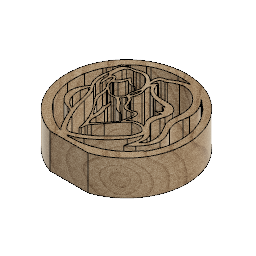
mother's-day-01-v2 (Autodesk Fusion 360 design; units mm, degrees)
Autodesk Fusion 360 part; units mm, degrees
(part 1 of 2)
sketch "Sketch1" plane through (0, 0, 0) normal (0, 0, 1) x (1, 0, 0)
  spline S0 degree 3 poles (69.4054, 110.167) (64.1585, 109.9181) (58.2066, 108.342) (54.0588, 106.0815) knots 0 0 0 0 1 1 1 1
  spline S1 degree 3 poles (54.0588, 106.0815) (53.4367, 105.7289) (52.5034, 105.2312) (51.985, 104.9409) knots 0 0 0 0 1 1 1 1
  spline S2 degree 3 poles (51.985, 104.9409) (49.1438, 103.4062) (45.3279, 100.4198) (45.5145, 99.8599) knots 0 0 0 0 1 1 1 1
  spline S3 degree 3 poles (45.5145, 99.8599) (45.5352, 99.7562) (45.4938, 99.7355) (45.3901, 99.7977) knots 0 0 0 0 1 1 1 1
  spline S4 degree 3 poles (45.3901, 99.7977) (45.2864, 99.8599) (44.9753, 99.6733) (44.7057, 99.3622) knots 0 0 0 0 1 1 1 1
  spline S5 degree 3 poles (44.7057, 99.3622) (44.3117, 98.9267) (44.2909, 98.8437) (44.5813, 98.9474) knots 0 0 0 0 1 1 1 1
  spline S6 degree 3 poles (44.5813, 98.9474) (44.8094, 99.0304) (44.9131, 99.0096) (44.8301, 98.8852) knots 0 0 0 0 1 1 1 1
  spline S7 degree 3 poles (44.8301, 98.8852) (44.7679, 98.7608) (44.5191, 98.6778) (44.2909, 98.6778) knots 0 0 0 0 1 1 1 1
  spline S8 degree 3 poles (44.2909, 98.6778) (43.8554, 98.6778) (43.7517, 98.3667) (44.1665, 98.1801) knots 0 0 0 0 1 1 1 1
  spline S9 degree 3 poles (44.1665, 98.1801) (44.2909, 98.1179) (44.1872, 98.1179) (43.8969, 98.1801) knots 0 0 0 0 1 1 1 1
  spline S10 degree 3 poles (43.8969, 98.1801) (43.4821, 98.263) (43.2125, 98.0971) (42.5696, 97.4542) knots 0 0 0 0 1 1 1 1
  spline S11 degree 3 poles (42.5696, 97.4542) (42.1341, 97.0187) (41.8438, 96.5417) (41.906, 96.4173) knots 0 0 0 0 1 1 1 1
  spline S12 degree 3 poles (41.906, 96.4173) (41.9889, 96.2929) (41.9267, 96.1892) (41.7816, 96.1892) knots 0 0 0 0 1 1 1 1
  spline S13 degree 3 poles (41.7816, 96.1892) (41.6364, 96.1892) (41.4912, 95.9196) (41.4705, 95.567) knots 0 0 0 0 1 1 1 1
  spline S14 degree 3 poles (41.4705, 95.567) (41.4497, 95.2352) (41.4083, 94.7789) (41.3875, 94.5923) knots 0 0 0 0 1 1 1 1
  spline S15 degree 3 poles (41.3875, 94.5923) (41.3668, 94.3849) (40.8691, 93.4724) (40.2676, 92.5599) knots 0 0 0 0 1 1 1 1
  spline S16 degree 3 poles (40.2676, 92.5599) (39.6662, 91.6474) (38.8781, 90.3409) (38.5048, 89.6565) knots 0 0 0 0 1 1 1 1
  spline S17 degree 3 poles (38.5048, 89.6565) (38.1316, 88.9721) (37.696, 88.2255) (37.5509, 87.9974) knots 0 0 0 0 1 1 1 1
  spline S18 degree 3 poles (37.5509, 87.9974) (36.6591, 86.5872) (35.1037, 81.838) (34.3156, 78.1051) knots 0 0 0 0 1 1 1 1
  spline S19 degree 3 poles (34.3156, 78.1051) (33.7142, 75.1809) (33.569, 69.4156) (34.0046, 66.2218) knots 0 0 0 0 1 1 1 1
  spline S20 degree 3 poles (34.0046, 66.2218) (34.9585, 59.5232) (36.7835, 54.5045) (39.8943, 50.1079) knots 0 0 0 0 1 1 1 1
  spline S21 degree 3 poles (39.8943, 50.1079) (42.8392, 45.9809) (49.7659, 39.8423) (54.3284, 37.3329) knots 0 0 0 0 1 1 1 1
  spline S22 degree 3 poles (54.3284, 37.3329) (56.4852, 36.1508) (60.4256, 34.471) (60.6122, 34.6576) knots 0 0 0 0 1 1 1 1
  spline S23 degree 3 poles (60.6122, 34.6576) (60.6952, 34.7198) (60.4463, 35.0931) (60.0938, 35.4664) knots 0 0 0 0 1 1 1 1
  spline S24 degree 3 poles (60.0938, 35.4664) (58.1443, 37.5403) (54.8884, 43.2227) (52.6901, 48.3866) knots 0 0 0 0 1 1 1 1
  spline S25 degree 3 poles (52.6901, 48.3866) (52.2131, 49.5272) (51.6946, 50.5227) (51.5287, 50.5849) knots 0 0 0 0 1 1 1 1
  spline S26 degree 3 poles (51.5287, 50.5849) (51.3835, 50.6678) (50.3466, 51.0204) (49.2267, 51.373) knots 0 0 0 0 1 1 1 1
  spline S27 degree 3 poles (49.2267, 51.373) (46.0537, 52.3684) (44.6227, 53.1565) (42.9637, 54.8156) knots 0 0 0 0 1 1 1 1
  spline S28 degree 3 poles (42.9637, 54.8156) (41.4497, 56.3502) (40.3713, 58.196) (39.8321, 60.2076) knots 0 0 0 0 1 1 1 1
  spline S29 degree 3 poles (39.8321, 60.2076) (38.9818, 63.3392) (40.081, 67.7565) (42.5696, 71.2198) knots 0 0 0 0 1 1 1 1
  spline S30 degree 3 poles (42.5696, 71.2198) (43.1503, 72.0286) (43.6895, 72.796) (43.7725, 72.9204) knots 0 0 0 0 1 1 1 1
  spline S31 degree 3 poles (43.7725, 72.9204) (43.8347, 73.0448) (43.6688, 73.4803) (43.3784, 73.8951) knots 0 0 0 0 1 1 1 1
  spline S32 degree 3 poles (43.3784, 73.8951) (41.0972, 77.2755) (40.3506, 81.9625) (41.4083, 86.442) knots 0 0 0 0 1 1 1 1
  spline S33 degree 3 poles (41.4083, 86.442) (41.6571, 87.5204) (41.9267, 89.6357) (42.0304, 91.1082) knots 0 0 0 0 1 1 1 1
  spline S34 degree 3 poles (42.0304, 91.1082) (42.2585, 95.1937) (42.8807, 96.2929) (45.7012, 97.7238) knots 0 0 0 0 1 1 1 1
  spline S35 degree 3 poles (45.7012, 97.7238) (46.9662, 98.346) (48.8534, 98.8852) (49.8489, 98.8852) knots 0 0 0 0 1 1 1 1
  spline S36 degree 3 poles (49.8489, 98.8852) (50.2429, 98.8852) (50.8858, 99.1133) (51.3421, 99.4036) knots 0 0 0 0 1 1 1 1
  spline S37 degree 3 poles (51.3421, 99.4036) (52.3168, 100.0673) (55.1995, 100.6272) (56.7134, 100.4821) knots 0 0 0 0 1 1 1 1
  spline S38 degree 3 poles (56.7134, 100.4821) (57.9992, 100.3369) (60.0523, 99.3) (61.6284, 97.9519) knots 0 0 0 0 1 1 1 1
  line L0 (61.6284, 97.9519) -> (62.6861, 97.0394)
  line L1 (62.6861, 97.0394) -> (62.6031, 98.3875)
  spline S39 degree 3 poles (62.6031, 98.3875) (62.3958, 101.5605) (63.9304, 103.5099) (67.0205, 103.9661) knots 0 0 0 0 1 1 1 1
  spline S40 degree 3 poles (67.0205, 103.9661) (67.7878, 104.0906) (68.3477, 104.3809) (69.4884, 105.2727) knots 0 0 0 0 1 1 1 1
  spline S41 degree 3 poles (69.4884, 105.2727) (71.8733, 107.1184) (76.8506, 109.2545) (78.8, 109.2545) knots 0 0 0 0 1 1 1 1
  spline S42 degree 3 poles (78.8, 109.2545) (79.5259, 109.2545) (79.0074, 109.5034) (77.6594, 109.7937) knots 0 0 0 0 1 1 1 1
  spline S43 degree 3 poles (77.6594, 109.7937) (76.2906, 110.1048) (72.0185, 110.2914) (69.4054, 110.167) knots 0 0 0 0 1 1 1 1
  spline S44 degree 3 poles (41.823, 94.7375) (41.823, 94.6338) (41.7193, 94.5301) (41.5949, 94.5301) knots 0 0 0 0 1 1 1 1
  spline S45 degree 3 poles (41.5949, 94.5301) (41.4912, 94.5301) (41.4497, 94.6338) (41.5119, 94.7375) knots 0 0 0 0 1 1 1 1
  spline S46 degree 3 poles (41.5119, 94.7375) (41.5742, 94.8619) (41.6779, 94.9448) (41.7401, 94.9448) knots 0 0 0 0 1 1 1 1
  spline S47 degree 3 poles (41.7401, 94.9448) (41.7816, 94.9448) (41.823, 94.8619) (41.823, 94.7375) knots 0 0 0 0 1 1 1 1
  spline S48 degree 3 poles (75.2952, 105.4386) (73.4287, 104.8372) (70.5253, 103.261) (69.7372, 102.4315) knots 0 0 0 0 1 1 1 1
  spline S49 degree 3 poles (69.7372, 102.4315) (69.3225, 101.996) (68.9284, 101.8093) (68.4929, 101.7886) knots 0 0 0 0 1 1 1 1
  spline S50 degree 3 poles (68.4929, 101.7886) (67.2279, 101.7679) (66.9997, 101.7264) (66.1702, 101.2494) knots 0 0 0 0 1 1 1 1
  spline S51 degree 3 poles (66.1702, 101.2494) (65.4651, 100.8346) (65.2577, 100.5443) (64.9674, 99.6525) knots 0 0 0 0 1 1 1 1
  spline S52 degree 3 poles (64.9674, 99.6525) (64.76, 99.0718) (64.5526, 97.869) (64.5111, 97.0187) knots 0 0 0 0 1 1 1 1
  line L2 (64.5111, 97.0187) -> (64.4074, 95.4633)
  line L3 (64.4074, 95.4633) -> (64.8844, 96.0855)
  spline S53 degree 3 poles (64.8844, 96.0855) (65.631, 97.0602) (66.9583, 98.4704) (67.1242, 98.4704) knots 0 0 0 0 1 1 1 1
  spline S54 degree 3 poles (67.1242, 98.4704) (67.2071, 98.4704) (67.3316, 98.0142) (67.4145, 97.4542) knots 0 0 0 0 1 1 1 1
  spline S55 degree 3 poles (67.4145, 97.4542) (67.5804, 96.1684) (68.7625, 93.7835) (69.7165, 92.8088) knots 0 0 0 0 1 1 1 1
  spline S56 degree 3 poles (69.7165, 92.8088) (70.7327, 91.7718) (72.06, 91.0252) (73.8227, 90.5275) knots 0 0 0 0 1 1 1 1
  spline S57 degree 3 poles (73.8227, 90.5275) (75.0878, 90.175) (76.021, 90.1127) (79.9821, 90.0713) knots 0 0 0 0 1 1 1 1
  spline S58 degree 3 poles (79.9821, 90.0713) (82.5537, 90.0505) (84.9387, 89.9261) (85.2912, 89.8224) knots 0 0 0 0 1 1 1 1
  spline S59 degree 3 poles (85.2912, 89.8224) (87.925, 88.9306) (89.7915, 87.313) (90.4137, 85.4051) knots 0 0 0 0 1 1 1 1
  spline S60 degree 3 poles (90.4137, 85.4051) (90.8907, 83.9119) (90.8699, 81.4232) (90.3722, 79.9923) knots 0 0 0 0 1 1 1 1
  spline S61 degree 3 poles (90.3722, 79.9923) (90.1441, 79.3701) (89.7085, 78.1673) (89.3975, 77.317) knots 0 0 0 0 1 1 1 1
  spline S62 degree 3 poles (89.3975, 77.317) (88.6509, 75.2639) (88.485, 72.6508) (89.0034, 71.0954) knots 0 0 0 0 1 1 1 1
  spline S63 degree 3 poles (89.0034, 71.0954) (89.3767, 69.9548) (89.8537, 69.4363) (94.3125, 65.1849) knots 0 0 0 0 1 1 1 1
  spline S64 degree 3 poles (94.3125, 65.1849) (96.3242, 63.2769) (96.9463, 62.1985) (97.2574, 60.021) knots 0 0 0 0 1 1 1 1
  spline S65 degree 3 poles (97.2574, 60.021) (97.4233, 58.8181) (97.4026, 58.1752) (97.133, 56.6821) knots 0 0 0 0 1 1 1 1
  spline S66 degree 3 poles (97.133, 56.6821) (96.9463, 55.6659) (96.8219, 54.8156) (96.8426, 54.7741) knots 0 0 0 0 1 1 1 1
  spline S67 degree 3 poles (96.8426, 54.7741) (96.9463, 54.6704) (98.7921, 56.4747) (99.1446, 57.0139) knots 0 0 0 0 1 1 1 1
  spline S68 degree 3 poles (99.1446, 57.0139) (99.9534, 58.2997) (100.4926, 61.1201) (100.2438, 63.0073) knots 0 0 0 0 1 1 1 1
  spline S69 degree 3 poles (100.2438, 63.0073) (100.1401, 63.7539) (100.0779, 64.6249) (100.0779, 64.936) knots 0 0 0 0 1 1 1 1
  spline S70 degree 3 poles (100.0779, 64.936) (100.0779, 65.4338) (100.0364, 65.496) (99.7875, 65.2886) knots 0 0 0 0 1 1 1 1
  spline S71 degree 3 poles (99.7875, 65.2886) (99.435, 64.9982) (99.3728, 65.2264) (99.6838, 65.7034) knots 0 0 0 0 1 1 1 1
  spline S72 degree 3 poles (99.6838, 65.7034) (99.7875, 65.8693) (99.7875, 66.0974) (99.7046, 66.2218) knots 0 0 0 0 1 1 1 1
  spline S73 degree 3 poles (99.7046, 66.2218) (99.6009, 66.3255) (99.4764, 66.6988) (99.3935, 67.0514) knots 0 0 0 0 1 1 1 1
  spline S74 degree 3 poles (99.3935, 67.0514) (99.3105, 67.3832) (99.1239, 67.798) (98.9995, 67.9639) knots 0 0 0 0 1 1 1 1
  spline S75 degree 3 poles (98.9995, 67.9639) (98.8543, 68.1298) (98.7506, 68.3994) (98.7506, 68.586) knots 0 0 0 0 1 1 1 1
  spline S76 degree 3 poles (98.7506, 68.586) (98.7506, 69.063) (96.9256, 72.5264) (96.7389, 72.4227) knots 0 0 0 0 1 1 1 1
  spline S77 degree 3 poles (96.7389, 72.4227) (96.656, 72.3605) (96.573, 72.4642) (96.573, 72.6301) knots 0 0 0 0 1 1 1 1
  spline S78 degree 3 poles (96.573, 72.6301) (96.573, 72.8167) (96.4693, 72.9619) (96.3449, 72.9619) knots 0 0 0 0 1 1 1 1
  spline S79 degree 3 poles (96.3449, 72.9619) (96.2412, 72.9619) (96.179, 73.0448) (96.2412, 73.1485) knots 0 0 0 0 1 1 1 1
  spline S80 degree 3 poles (96.2412, 73.1485) (96.3034, 73.2522) (96.179, 73.5426) (95.9716, 73.8122) knots 0 0 0 0 1 1 1 1
  spline S81 degree 3 poles (95.9716, 73.8122) (94.831, 75.2846) (93.8978, 78.2502) (93.8563, 80.6352) knots 0 0 0 0 1 1 1 1
  spline S82 degree 3 poles (93.8563, 80.6352) (93.8355, 81.4855) (93.9392, 83.7875) (94.0844, 85.7161) knots 0 0 0 0 1 1 1 1
  spline S83 degree 3 poles (94.0844, 85.7161) (94.3333, 88.9099) (94.3125, 89.4491) (94.0014, 91.4193) knots 0 0 0 0 1 1 1 1
  spline S84 degree 3 poles (94.0014, 91.4193) (93.4622, 94.5508) (92.612, 96.7491) (91.1603, 98.6778) knots 0 0 0 0 1 1 1 1
  spline S85 degree 3 poles (91.1603, 98.6778) (86.7429, 104.5261) (80.5835, 107.1599) (75.2952, 105.4386) knots 0 0 0 0 1 1 1 1
  spline S86 degree 3 poles (93.3378, 102.7633) (96.9878, 99.0511) (99.0617, 93.8042) (98.7713, 89.0965) knots 0 0 0 0 1 1 1 1
  spline S87 degree 3 poles (98.7713, 89.0965) (98.7091, 87.9974) (98.4603, 86.1309) (98.2114, 84.9488) knots 0 0 0 0 1 1 1 1
  spline S88 degree 3 poles (98.2114, 84.9488) (97.3404, 80.5522) (97.8588, 77.0889) (99.912, 73.584) knots 0 0 0 0 1 1 1 1
  spline S89 degree 3 poles (99.912, 73.584) (102.608, 69.0215) (103.6242, 66.1389) (103.6242, 63.1525) knots 0 0 0 0 1 1 1 1
  spline S90 degree 3 poles (103.6242, 63.1525) (103.6242, 59.3988) (101.8614, 55.811) (97.8588, 51.4144) knots 0 0 0 0 1 1 1 1
  spline S91 degree 3 poles (97.8588, 51.4144) (96.5108, 49.942) (93.3585, 47.2874) (93.1512, 47.4741) knots 0 0 0 0 1 1 1 1
  spline S92 degree 3 poles (93.1512, 47.4741) (93.1097, 47.5156) (93.3585, 48.4073) (93.6904, 49.4235) knots 0 0 0 0 1 1 1 1
  spline S93 degree 3 poles (93.6904, 49.4235) (95.5154, 54.9815) (95.6191, 58.8596) (94.0014, 60.8298) knots 0 0 0 0 1 1 1 1
  line L4 (94.0014, 60.8298) -> (93.483, 61.4519)
  line L5 (93.483, 61.4519) -> (93.4622, 60.7053)
  spline S94 degree 3 poles (93.4622, 60.7053) (93.4622, 59.1292) (92.1142, 55.9562) (90.2063, 53.0113) knots 0 0 0 0 1 1 1 1
  spline S95 degree 3 poles (90.2063, 53.0113) (87.054, 48.0963) (80.5421, 41.7502) (74.4656, 37.6647) knots 0 0 0 0 1 1 1 1
  spline S96 degree 3 poles (74.4656, 37.6647) (71.9355, 35.9641) (70.8364, 35.4042) (68.6796, 34.6991) knots 0 0 0 0 1 1 1 1
  spline S97 degree 3 poles (68.6796, 34.6991) (66.1702, 33.8695) (65.9628, 33.7659) (66.2946, 33.5585) knots 0 0 0 0 1 1 1 1
  spline S98 degree 3 poles (66.2946, 33.5585) (66.7924, 33.2474) (69.8824, 33.3303) (73.6983, 33.7451) knots 0 0 0 0 1 1 1 1
  spline S99 degree 3 poles (73.6983, 33.7451) (77.2031, 34.1391) (77.7009, 34.2428) (80.3969, 35.0102) knots 0 0 0 0 1 1 1 1
  spline S100 degree 3 poles (80.3969, 35.0102) (81.1435, 35.2383) (81.9938, 35.4664) (82.3049, 35.5494) knots 0 0 0 0 1 1 1 1
  spline S101 degree 3 poles (82.3049, 35.5494) (82.6367, 35.6116) (82.8233, 35.7568) (82.7611, 35.8605) knots 0 0 0 0 1 1 1 1
  spline S102 degree 3 poles (82.7611, 35.8605) (82.6989, 35.9641) (82.7818, 35.9849) (82.9478, 35.9434) knots 0 0 0 0 1 1 1 1
  spline S103 degree 3 poles (82.9478, 35.9434) (83.3003, 35.7982) (86.0585, 36.9596) (85.8512, 37.167) knots 0 0 0 0 1 1 1 1
  spline S104 degree 3 poles (85.8512, 37.167) (85.7682, 37.2499) (85.8512, 37.2499) (86.0171, 37.1877) knots 0 0 0 0 1 1 1 1
  spline S105 degree 3 poles (86.0171, 37.1877) (86.5563, 36.9803) (91.0151, 39.4275) (93.6904, 41.3769) knots 0 0 0 0 1 1 1 1
  spline S106 degree 3 poles (93.6904, 41.3769) (96.9256, 43.7411) (99.6424, 46.3749) (101.8407, 49.3198) knots 0 0 0 0 1 1 1 1
  spline S107 degree 3 poles (101.8407, 49.3198) (103.1679, 51.0619) (103.7693, 51.6633) (103.8938, 51.3315) knots 0 0 0 0 1 1 1 1
  spline S108 degree 3 poles (103.8938, 51.3315) (103.956, 51.1863) (104.0182, 51.2278) (104.0182, 51.4144) knots 0 0 0 0 1 1 1 1
  spline S109 degree 3 poles (104.0182, 51.4144) (104.0389, 51.6011) (104.1634, 51.8085) (104.3086, 51.8707) knots 0 0 0 0 1 1 1 1
  spline S110 degree 3 poles (104.3086, 51.8707) (104.433, 51.9122) (104.7441, 52.3269) (104.9929, 52.7624) knots 0 0 0 0 1 1 1 1
  spline S111 degree 3 poles (104.9929, 52.7624) (105.2211, 53.2187) (105.7395, 54.1312) (106.1128, 54.8156) knots 0 0 0 0 1 1 1 1
  spline S112 degree 3 poles (106.1128, 54.8156) (107.9171, 58.1545) (109.5347, 63.7539) (109.8665, 67.9639) knots 0 0 0 0 1 1 1 1
  spline S113 degree 3 poles (109.8665, 67.9639) (110.2191, 72.4434) (109.8043, 77.3377) (108.7051, 81.5269) knots 0 0 0 0 1 1 1 1
  spline S114 degree 3 poles (108.7051, 81.5269) (108.1452, 83.663) (106.258, 88.3707) (105.1588, 90.3201) knots 0 0 0 0 1 1 1 1
  spline S115 degree 3 poles (105.1588, 90.3201) (104.433, 91.6267) (101.0111, 96.2721) (99.8083, 97.5786) knots 0 0 0 0 1 1 1 1
  spline S116 degree 3 poles (99.8083, 97.5786) (99.4557, 97.9727) (99.0824, 98.4289) (98.9995, 98.5948) knots 0 0 0 0 1 1 1 1
  spline S117 degree 3 poles (98.9995, 98.5948) (98.9165, 98.7608) (98.7299, 98.8852) (98.5847, 98.8852) knots 0 0 0 0 1 1 1 1
  spline S118 degree 3 poles (98.5847, 98.8852) (98.4395, 98.8852) (98.2114, 99.0718) (98.0662, 99.3) knots 0 0 0 0 1 1 1 1
  spline S119 degree 3 poles (98.0662, 99.3) (97.921, 99.5281) (97.6307, 99.7147) (97.3818, 99.7147) knots 0 0 0 0 1 1 1 1
  spline S120 degree 3 poles (97.3818, 99.7147) (97.1537, 99.7147) (97.0085, 99.7977) (97.0915, 99.9014) knots 0 0 0 0 1 1 1 1
  spline S121 degree 3 poles (97.0915, 99.9014) (97.1537, 100.0258) (97.0293, 100.2125) (96.8219, 100.3161) knots 0 0 0 0 1 1 1 1
  spline S122 degree 3 poles (96.8219, 100.3161) (96.5938, 100.4406) (96.0131, 100.9383) (95.5154, 101.436) knots 0 0 0 0 1 1 1 1
  spline S123 degree 3 poles (95.5154, 101.436) (94.6651, 102.2863) (92.4046, 104.0698) (92.1764, 104.0698) knots 0 0 0 0 1 1 1 1
  spline S124 degree 3 poles (92.1764, 104.0698) (92.135, 104.0698) (92.6534, 103.4892) (93.3378, 102.7633) knots 0 0 0 0 1 1 1 1
  spline S125 degree 3 poles (53.9551, 98.2838) (53.3745, 98.1801) (52.5034, 97.9105) (52.0057, 97.6409) knots 0 0 0 0 1 1 1 1
  spline S126 degree 3 poles (52.0057, 97.6409) (51.3421, 97.309) (50.8858, 97.2261) (50.3466, 97.309) knots 0 0 0 0 1 1 1 1
  spline S127 degree 3 poles (50.3466, 97.309) (49.1645, 97.4957) (47.4639, 96.9358) (46.6137, 96.1062) knots 0 0 0 0 1 1 1 1
  spline S128 degree 3 poles (46.6137, 96.1062) (46.0122, 95.5255) (45.7841, 95.0693) (45.5145, 93.8664) knots 0 0 0 0 1 1 1 1
  spline S129 degree 3 poles (45.5145, 93.8664) (44.9546, 91.5644) (44.7057, 89.4491) (44.8509, 88.2048) knots 0 0 0 0 1 1 1 1
  line L6 (44.8509, 88.2048) -> (44.996, 87.0849)
  line L7 (44.996, 87.0849) -> (45.5145, 87.4789)
  spline S130 degree 3 poles (45.5145, 87.4789) (46.6137, 88.35) (47.9824, 87.6863) (48.7705, 85.8821) knots 0 0 0 0 1 1 1 1
  spline S131 degree 3 poles (48.7705, 85.8821) (48.9364, 85.5088) (49.1438, 85.1977) (49.2267, 85.1977) knots 0 0 0 0 1 1 1 1
  spline S132 degree 3 poles (49.2267, 85.1977) (49.7867, 85.1977) (50.8858, 86.7116) (52.0887, 89.1588) knots 0 0 0 0 1 1 1 1
  spline S133 degree 3 poles (52.0887, 89.1588) (52.8352, 90.6519) (53.4367, 92.0207) (53.4367, 92.1659) knots 0 0 0 0 1 1 1 1
  spline S134 degree 3 poles (53.4367, 92.1659) (53.4367, 92.3318) (53.4781, 92.4562) (53.5196, 92.4562) knots 0 0 0 0 1 1 1 1
  spline S135 degree 3 poles (53.5196, 92.4562) (53.5611, 92.4562) (54.287, 91.7718) (55.1165, 90.9423) knots 0 0 0 0 1 1 1 1
  spline S136 degree 3 poles (55.1165, 90.9423) (56.7963, 89.3039) (58.0821, 88.5573) (59.8656, 88.184) knots 0 0 0 0 1 1 1 1
  spline S137 degree 3 poles (59.8656, 88.184) (60.6537, 88.0389) (61.027, 87.8522) (61.0685, 87.6241) knots 0 0 0 0 1 1 1 1
  spline S138 degree 3 poles (61.0685, 87.6241) (61.11, 87.4167) (61.0063, 87.2715) (60.8196, 87.2715) knots 0 0 0 0 1 1 1 1
  spline S139 degree 3 poles (60.8196, 87.2715) (60.633, 87.2715) (60.4878, 87.3545) (60.4878, 87.4582) knots 0 0 0 0 1 1 1 1
  spline S140 degree 3 poles (60.4878, 87.4582) (60.4878, 87.5619) (59.679, 87.6863) (58.6835, 87.7278) knots 0 0 0 0 1 1 1 1
  spline S141 degree 3 poles (58.6835, 87.7278) (56.7548, 87.8315) (56.3193, 87.9974) (54.9506, 89.0758) knots 0 0 0 0 1 1 1 1
  line L8 (54.9506, 89.0758) -> (54.1003, 89.7602)
  line L9 (54.1003, 89.7602) -> (53.7685, 88.3914)
  spline S142 degree 3 poles (53.7685, 88.3914) (53.25, 86.3176) (52.5034, 84.9696) (51.7776, 84.8244) knots 0 0 0 0 1 1 1 1
  spline S143 degree 3 poles (51.7776, 84.8244) (51.2798, 84.7207) (50.0977, 83.4764) (50.2222, 83.1653) knots 0 0 0 0 1 1 1 1
  spline S144 degree 3 poles (50.2222, 83.1653) (50.2637, 83.0201) (50.2222, 82.9579) (50.1185, 83.0201) knots 0 0 0 0 1 1 1 1
  spline S145 degree 3 poles (50.1185, 83.0201) (49.9941, 83.0823) (49.9111, 82.9994) (49.9111, 82.8335) knots 0 0 0 0 1 1 1 1
  spline S146 degree 3 poles (49.9111, 82.8335) (49.9111, 82.6261) (49.7867, 82.5639) (49.6, 82.6261) knots 0 0 0 0 1 1 1 1
  spline S147 degree 3 poles (49.6, 82.6261) (49.206, 82.792) (49.206, 82.8127) (49.7037, 81.2366) knots 0 0 0 0 1 1 1 1
  spline S148 degree 3 poles (49.7037, 81.2366) (50.16, 79.7642) (51.1139, 78.6028) (52.4412, 77.9184) knots 0 0 0 0 1 1 1 1
  spline S149 degree 3 poles (52.4412, 77.9184) (52.856, 77.711) (53.7063, 77.0889) (54.287, 76.5704) knots 0 0 0 0 1 1 1 1
  spline S150 degree 3 poles (54.287, 76.5704) (54.8884, 76.0312) (55.6764, 75.4713) (56.0497, 75.3261) knots 0 0 0 0 1 1 1 1
  spline S151 degree 3 poles (56.0497, 75.3261) (57.5014, 74.7247) (59.5753, 75.098) (60.3219, 76.1142) knots 0 0 0 0 1 1 1 1
  spline S152 degree 3 poles (60.3219, 76.1142) (60.5915, 76.4667) (61.1307, 77.0889) (61.5455, 77.5036) knots 0 0 0 0 1 1 1 1
  spline S153 degree 3 poles (61.5455, 77.5036) (62.7691, 78.7272) (62.8313, 78.9968) (62.6861, 81.5477) knots 0 0 0 0 1 1 1 1
  spline S154 degree 3 poles (62.6861, 81.5477) (62.5617, 83.5801) (62.6031, 83.9534) (62.9557, 84.7) knots 0 0 0 0 1 1 1 1
  spline S155 degree 3 poles (62.9557, 84.7) (63.4327, 85.6954) (63.8889, 88.7232) (63.7023, 89.7394) knots 0 0 0 0 1 1 1 1
  spline S156 degree 3 poles (63.7023, 89.7394) (63.1216, 93.1198) (60.7989, 96.4173) (58.1236, 97.6616) knots 0 0 0 0 1 1 1 1
  spline S157 degree 3 poles (58.1236, 97.6616) (56.6926, 98.346) (55.4691, 98.5119) (53.9551, 98.2838) knots 0 0 0 0 1 1 1 1
  spline S158 degree 3 poles (65.9213, 93.5554) (65.5895, 92.7051) (65.8176, 90.486) (66.3776, 89.138) knots 0 0 0 0 1 1 1 1
  spline S159 degree 3 poles (66.3776, 89.138) (66.6679, 88.4122) (66.979, 87.3338) (67.0412, 86.7531) knots 0 0 0 0 1 1 1 1
  spline S160 degree 3 poles (67.0412, 86.7531) (67.2071, 85.3221) (66.8338, 82.8542) (66.1909, 81.2988) knots 0 0 0 0 1 1 1 1
  spline S161 degree 3 poles (66.1909, 81.2988) (65.6102, 79.8471) (65.7139, 79.3909) (66.6264, 79.3909) knots 0 0 0 0 1 1 1 1
  spline S162 degree 3 poles (66.6264, 79.3909) (67.1449, 79.3909) (67.7463, 78.5198) (67.7463, 77.7732) knots 0 0 0 0 1 1 1 1
  spline S163 degree 3 poles (67.7463, 77.7732) (67.7463, 77.5451) (68.0159, 77.0267) (68.3477, 76.6119) knots 0 0 0 0 1 1 1 1
  spline S164 degree 3 poles (68.3477, 76.6119) (68.6796, 76.1971) (69.0321, 75.5542) (69.0943, 75.1809) knots 0 0 0 0 1 1 1 1
  spline S165 degree 3 poles (69.0943, 75.1809) (69.7372, 72.0909) (71.8733, 71.1369) (75.2952, 72.4227) knots 0 0 0 0 1 1 1 1
  spline S166 degree 3 poles (75.2952, 72.4227) (76.498, 72.8789) (76.8506, 72.9411) (77.4105, 72.7545) knots 0 0 0 0 1 1 1 1
  spline S167 degree 3 poles (77.4105, 72.7545) (78.9452, 72.236) (79.3392, 70.8673) (78.8622, 67.6321) knots 0 0 0 0 1 1 1 1
  spline S168 degree 3 poles (78.8622, 67.6321) (78.3645, 64.2931) (78.3438, 64.0443) (78.4682, 64.0443) knots 0 0 0 0 1 1 1 1
  spline S169 degree 3 poles (78.4682, 64.0443) (78.5304, 64.0443) (79.0696, 64.459) (79.671, 64.9775) knots 0 0 0 0 1 1 1 1
  spline S170 degree 3 poles (79.671, 64.9775) (81.2679, 66.3463) (83.5906, 67.2173) (85.5816, 67.1965) knots 0 0 0 0 1 1 1 1
  spline S171 degree 3 poles (85.5816, 67.1965) (86.4318, 67.1965) (87.3858, 67.0928) (87.6969, 66.9684) knots 0 0 0 0 1 1 1 1
  line L10 (87.6969, 66.9684) -> (88.2776, 66.7403)
  line L11 (88.2776, 66.7403) -> (87.5725, 67.7772)
  spline S172 degree 3 poles (87.5725, 67.7772) (86.0793, 69.9548) (85.1668, 72.4849) (85.1668, 74.4758) knots 0 0 0 0 1 1 1 1
  spline S173 degree 3 poles (85.1668, 74.4758) (85.1668, 75.5335) (85.7267, 77.3792) (86.6185, 79.2457) knots 0 0 0 0 1 1 1 1
  spline S174 degree 3 poles (86.6185, 79.2457) (86.9918, 80.013) (87.2406, 80.6974) (87.1992, 80.7596) knots 0 0 0 0 1 1 1 1
  spline S175 degree 3 poles (87.1992, 80.7596) (87.137, 80.8011) (86.7844, 80.6767) (86.3904, 80.49) knots 0 0 0 0 1 1 1 1
  spline S176 degree 3 poles (86.3904, 80.49) (85.4364, 80.013) (82.8855, 79.8471) (82.8855, 80.2619) knots 0 0 0 0 1 1 1 1
  spline S177 degree 3 poles (82.8855, 80.2619) (82.8855, 80.4485) (83.2381, 80.6767) (83.7151, 80.8218) knots 0 0 0 0 1 1 1 1
  spline S178 degree 3 poles (83.7151, 80.8218) (84.9594, 81.1951) (85.7889, 81.9832) (85.7889, 82.8127) knots 0 0 0 0 1 1 1 1
  spline S179 degree 3 poles (85.7889, 82.8127) (85.7889, 83.7252) (84.8764, 84.7) (83.8603, 84.8866) knots 0 0 0 0 1 1 1 1
  spline S180 degree 3 poles (83.8603, 84.8866) (83.4455, 84.9696) (83.0929, 85.0732) (83.0929, 85.1355) knots 0 0 0 0 1 1 1 1
  spline S181 degree 3 poles (83.0929, 85.1355) (83.0929, 85.1977) (83.2796, 85.488) (83.5284, 85.7784) knots 0 0 0 0 1 1 1 1
  line L12 (83.5284, 85.7784) -> (83.9639, 86.3383)
  line L13 (83.9639, 86.3383) -> (82.3256, 86.4835)
  spline S182 degree 3 poles (82.3256, 86.4835) (79.2563, 86.7738) (77.3483, 87.0642) (75.8759, 87.4582) knots 0 0 0 0 1 1 1 1
  spline S183 degree 3 poles (75.8759, 87.4582) (74.8389, 87.7278) (74.3827, 87.7693) (74.3827, 87.6034) knots 0 0 0 0 1 1 1 1
  spline S184 degree 3 poles (74.3827, 87.6034) (74.3827, 87.4789) (74.279, 87.5411) (74.1546, 87.7485) knots 0 0 0 0 1 1 1 1
  spline S185 degree 3 poles (74.1546, 87.7485) (74.0509, 87.9352) (73.8227, 88.1011) (73.6776, 88.1011) knots 0 0 0 0 1 1 1 1
  spline S186 degree 3 poles (73.6776, 88.1011) (73.1176, 88.1011) (70.0483, 89.7602) (68.9492, 90.6934) knots 0 0 0 0 1 1 1 1
  spline S187 degree 3 poles (68.9492, 90.6934) (68.2855, 91.2326) (67.4352, 92.1659) (67.0205, 92.788) knots 0 0 0 0 1 1 1 1
  spline S188 degree 3 poles (67.0205, 92.788) (66.6057, 93.4102) (66.2324, 93.9079) (66.1702, 93.9079) knots 0 0 0 0 1 1 1 1
  spline S189 degree 3 poles (66.1702, 93.9079) (66.1287, 93.9079) (66.0043, 93.742) (65.9213, 93.5554) knots 0 0 0 0 1 1 1 1
  spline S190 degree 3 poles (65.0088, 86.7116) (64.8222, 85.9028) (64.4281, 84.7414) (64.1378, 84.1193) knots 0 0 0 0 1 1 1 1
  spline S191 degree 3 poles (64.1378, 84.1193) (63.5986, 82.9994) (63.4949, 82.1284) (63.7645, 81.4232) knots 0 0 0 0 1 1 1 1
  spline S192 degree 3 poles (63.7645, 81.4232) (63.9926, 80.8426) (64.3659, 81.2781) (64.9259, 82.709) knots 0 0 0 0 1 1 1 1
  spline S193 degree 3 poles (64.9259, 82.709) (65.5273, 84.3267) (65.7554, 86.0065) (65.5273, 87.2508) knots 0 0 0 0 1 1 1 1
  line L14 (65.5273, 87.2508) -> (65.3614, 88.1633)
  line L15 (65.3614, 88.1633) -> (65.0088, 86.7116)
  spline S194 degree 3 poles (42.9222, 83.6008) (43.0259, 79.9093) (43.4199, 77.5451) (44.1872, 76.0934) knots 0 0 0 0 1 1 1 1
  spline S195 degree 3 poles (44.1872, 76.0934) (45.3901, 73.7914) (45.7634, 73.1693) (46.6137, 72.2568) knots 0 0 0 0 1 1 1 1
  spline S196 degree 3 poles (46.6137, 72.2568) (48.3557, 70.3281) (49.1852, 68.192) (50.8443, 61.3897) knots 0 0 0 0 1 1 1 1
  spline S197 degree 3 poles (50.8443, 61.3897) (52.2338, 55.6659) (53.4159, 52.3684) (55.6557, 47.8681) knots 0 0 0 0 1 1 1 1
  spline S198 degree 3 poles (55.6557, 47.8681) (58.3102, 42.5176) (61.1514, 38.2247) (62.6861, 37.1877) knots 0 0 0 0 1 1 1 1
  spline S199 degree 3 poles (62.6861, 37.1877) (63.5156, 36.6278) (64.9051, 36.5656) (66.2117, 37.0011) knots 0 0 0 0 1 1 1 1
  spline S200 degree 3 poles (66.2117, 37.0011) (68.2648, 37.6855) (73.3872, 40.5474) (73.8435, 41.2732) knots 0 0 0 0 1 1 1 1
  spline S201 degree 3 poles (73.8435, 41.2732) (73.9679, 41.4806) (74.1753, 41.6465) (74.2997, 41.6465) knots 0 0 0 0 1 1 1 1
  spline S202 degree 3 poles (74.2997, 41.6465) (74.6108, 41.6465) (77.9083, 44.1144) (77.9083, 44.3426) knots 0 0 0 0 1 1 1 1
  spline S203 degree 3 poles (77.9083, 44.3426) (77.9083, 44.4463) (78.0742, 44.5707) (78.2816, 44.6329) knots 0 0 0 0 1 1 1 1
  spline S204 degree 3 poles (78.2816, 44.6329) (79.0696, 44.9025) (84.752, 50.7923) (88.879, 55.6451) knots 0 0 0 0 1 1 1 1
  spline S205 degree 3 poles (88.879, 55.6451) (89.9159, 56.8894) (90.9736, 59.938) (90.9736, 61.763) knots 0 0 0 0 1 1 1 1
  spline S206 degree 3 poles (90.9736, 61.763) (90.9736, 62.5718) (90.8492, 62.8622) (90.2478, 63.5673) knots 0 0 0 0 1 1 1 1
  spline S207 degree 3 poles (90.2478, 63.5673) (88.402, 65.7241) (84.6691, 66.2426) (81.7034, 64.7286) knots 0 0 0 0 1 1 1 1
  spline S208 degree 3 poles (81.7034, 64.7286) (80.1895, 63.9821) (77.7009, 61.1201) (72.5162, 54.1934) knots 0 0 0 0 1 1 1 1
  spline S209 degree 3 poles (72.5162, 54.1934) (70.9816, 52.1403) (69.1566, 49.7346) (68.4307, 48.8428) knots 0 0 0 0 1 1 1 1
  line L16 (68.4307, 48.8428) -> (67.1449, 47.246)
  line L17 (67.1449, 47.246) -> (67.1656, 45.732)
  spline S210 degree 3 poles (67.1656, 45.732) (67.1864, 44.5707) (67.1034, 44.0522) (66.7509, 43.3678) knots 0 0 0 0 1 1 1 1
  spline S211 degree 3 poles (66.7509, 43.3678) (66.4813, 42.8701) (66.2117, 42.4761) (66.108, 42.4761) knots 0 0 0 0 1 1 1 1
  spline S212 degree 3 poles (66.108, 42.4761) (66.0043, 42.4761) (65.7762, 43.3056) (65.5895, 44.3218) knots 0 0 0 0 1 1 1 1
  spline S213 degree 3 poles (65.5895, 44.3218) (64.9881, 47.5156) (64.2415, 49.7346) (62.6654, 52.9491) knots 0 0 0 0 1 1 1 1
  spline S214 degree 3 poles (62.6654, 52.9491) (60.6745, 57.0346) (59.285, 59.1707) (56.8378, 61.9289) knots 0 0 0 0 1 1 1 1
  spline S215 degree 3 poles (56.8378, 61.9289) (54.4943, 64.5627) (53.1463, 66.3463) (52.5449, 67.5698) knots 0 0 0 0 1 1 1 1
  spline S216 degree 3 poles (52.5449, 67.5698) (51.9227, 68.8349) (51.8813, 69.063) (51.7568, 72.0286) knots 0 0 0 0 1 1 1 1
  spline S217 degree 3 poles (51.7568, 72.0286) (51.6117, 75.5957) (51.508, 75.9275) (49.4341, 79.1213) knots 0 0 0 0 1 1 1 1
  spline S218 degree 3 poles (49.4341, 79.1213) (48.1068, 81.1329) (47.6298, 82.5224) (47.6298, 84.2644) knots 0 0 0 0 1 1 1 1
  spline S219 degree 3 poles (47.6298, 84.2644) (47.6298, 85.6954) (47.2773, 86.2968) (46.6344, 85.9028) knots 0 0 0 0 1 1 1 1
  spline S220 degree 3 poles (46.6344, 85.9028) (46.1574, 85.5917) (45.8048, 83.3934) (45.9915, 81.921) knots 0 0 0 0 1 1 1 1
  spline S221 degree 3 poles (45.9915, 81.921) (46.0744, 81.2781) (46.1989, 79.9508) (46.2818, 78.9761) knots 0 0 0 0 1 1 1 1
  spline S222 degree 3 poles (46.2818, 78.9761) (46.427, 77.234) (46.427, 77.2133) (46.0122, 77.5866) knots 0 0 0 0 1 1 1 1
  spline S223 degree 3 poles (46.0122, 77.5866) (45.7841, 77.794) (45.3279, 78.5406) (45.0168, 79.2457) knots 0 0 0 0 1 1 1 1
  spline S224 degree 3 poles (45.0168, 79.2457) (44.4983, 80.3656) (44.4154, 80.7804) (44.4154, 82.5017) knots 0 0 0 0 1 1 1 1
  spline S225 degree 3 poles (44.4154, 82.5017) (44.4154, 84.2852) (44.3531, 84.5963) (43.731, 85.8821) knots 0 0 0 0 1 1 1 1
  spline S226 degree 3 poles (43.731, 85.8821) (43.3784, 86.6494) (43.0051, 87.2715) (42.9429, 87.2715) knots 0 0 0 0 1 1 1 1
  spline S227 degree 3 poles (42.9429, 87.2715) (42.86, 87.2715) (42.86, 85.6125) (42.9222, 83.6008) knots 0 0 0 0 1 1 1 1
  spline S228 degree 3 poles (63.8475, 78.1673) (63.7023, 77.711) (63.2668, 77.0681) (62.8105, 76.6741) knots 0 0 0 0 1 1 1 1
  spline S229 degree 3 poles (62.8105, 76.6741) (62.375, 76.2801) (61.9602, 75.8653) (61.8773, 75.7201) knots 0 0 0 0 1 1 1 1
  spline S230 degree 3 poles (61.8773, 75.7201) (61.7736, 75.5542) (62.2921, 75.0772) (63.4327, 74.3514) knots 0 0 0 0 1 1 1 1
  spline S231 degree 3 poles (63.4327, 74.3514) (65.3406, 73.1071) (65.6725, 72.7752) (66.9583, 70.971) knots 0 0 0 0 1 1 1 1
  spline S232 degree 3 poles (66.9583, 70.971) (67.9952, 69.5193) (69.758, 67.8602) (71.1889, 67.0306) knots 0 0 0 0 1 1 1 1
  line L18 (71.1889, 67.0306) -> (72.2051, 66.4292)
  line L19 (72.2051, 66.4292) -> (71.4585, 66.367)
  spline S233 degree 3 poles (71.4585, 66.367) (69.8617, 66.2218) (66.7509, 67.9639) (65.237, 69.8511) knots 0 0 0 0 1 1 1 1
  spline S234 degree 3 poles (65.237, 69.8511) (63.6816, 71.8005) (62.8105, 72.6508) (61.6284, 73.4181) knots 0 0 0 0 1 1 1 1
  spline S235 degree 3 poles (61.6284, 73.4181) (60.4878, 74.1855) (60.3219, 74.2269) (59.4509, 74.0818) knots 0 0 0 0 1 1 1 1
  spline S236 degree 3 poles (59.4509, 74.0818) (58.9324, 73.9988) (57.854, 73.9366) (57.0452, 73.9366) knots 0 0 0 0 1 1 1 1
  spline S237 degree 3 poles (57.0452, 73.9366) (55.3861, 73.9366) (54.7017, 74.2477) (53.4574, 75.5335) knots 0 0 0 0 1 1 1 1
  spline S238 degree 3 poles (53.4574, 75.5335) (53.0634, 75.9482) (52.6486, 76.2801) (52.5656, 76.2801) knots 0 0 0 0 1 1 1 1
  spline S239 degree 3 poles (52.5656, 76.2801) (52.462, 76.2801) (52.6486, 75.7823) (52.9597, 75.2017) knots 0 0 0 0 1 1 1 1
  spline S240 degree 3 poles (52.9597, 75.2017) (53.4159, 74.2892) (53.5404, 73.6877) (53.6648, 71.7383) knots 0 0 0 0 1 1 1 1
  spline S241 degree 3 poles (53.6648, 71.7383) (53.8722, 68.8971) (54.2247, 67.715) (55.4898, 65.8071) knots 0 0 0 0 1 1 1 1
  spline S242 degree 3 poles (55.4898, 65.8071) (56.8171, 63.7747) (62.5409, 56.1636) (62.7276, 56.1636) knots 0 0 0 0 1 1 1 1
  spline S243 degree 3 poles (62.7276, 56.1636) (62.9557, 56.1636) (62.6446, 59.4196) (62.2713, 60.9335) knots 0 0 0 0 1 1 1 1
  spline S244 degree 3 poles (62.2713, 60.9335) (62.0847, 61.6801) (61.7321, 62.717) (61.4833, 63.2562) knots 0 0 0 0 1 1 1 1
  spline S245 degree 3 poles (61.4833, 63.2562) (61.1307, 64.065) (61.0892, 64.3139) (61.2966, 64.8946) knots 0 0 0 0 1 1 1 1
  spline S246 degree 3 poles (61.2966, 64.8946) (61.6284, 65.8278) (61.587, 68.1505) (61.2137, 69.3534) knots 0 0 0 0 1 1 1 1
  spline S247 degree 3 poles (61.2137, 69.3534) (61.0477, 69.9133) (60.9026, 70.3903) (60.9026, 70.4318) knots 0 0 0 0 1 1 1 1
  spline S248 degree 3 poles (60.9026, 70.4318) (60.9026, 70.6806) (62.0017, 69.6644) (62.4372, 69.0423) knots 0 0 0 0 1 1 1 1
  spline S249 degree 3 poles (62.4372, 69.0423) (63.1631, 67.9846) (63.412, 67.0928) (63.412, 65.5374) knots 0 0 0 0 1 1 1 1
  spline S250 degree 3 poles (63.412, 65.5374) (63.3912, 64.4383) (63.5156, 63.9613) (64.1378, 62.6963) knots 0 0 0 0 1 1 1 1
  spline S251 degree 3 poles (64.1378, 62.6963) (65.0918, 60.7053) (65.2784, 59.4403) (65.237, 55.5414) knots 0 0 0 0 1 1 1 1
  spline S252 degree 3 poles (65.237, 55.5414) (65.1955, 52.721) (65.237, 52.161) (65.631, 50.9789) knots 0 0 0 0 1 1 1 1
  spline S253 degree 3 poles (65.631, 50.9789) (66.2531, 49.1539) (66.3776, 48.9673) (66.7924, 49.2991) knots 0 0 0 0 1 1 1 1
  spline S254 degree 3 poles (66.7924, 49.2991) (67.0412, 49.5065) (71.6867, 54.9815) (73.5739, 57.3042) knots 0 0 0 0 1 1 1 1
  spline S255 degree 3 poles (73.5739, 57.3042) (73.7813, 57.5323) (74.4864, 58.3826) (75.1915, 59.1914) knots 0 0 0 0 1 1 1 1
  spline S256 degree 3 poles (75.1915, 59.1914) (75.8759, 60.0002) (76.5395, 60.9335) (76.6639, 61.2653) knots 0 0 0 0 1 1 1 1
  spline S257 degree 3 poles (76.6639, 61.2653) (76.8713, 61.7838) (77.535, 65.7034) (77.846, 68.192) knots 0 0 0 0 1 1 1 1
  spline S258 degree 3 poles (77.846, 68.192) (77.9083, 68.7105) (77.846, 69.5193) (77.7216, 70.017) knots 0 0 0 0 1 1 1 1
  spline S259 degree 3 poles (77.7216, 70.017) (77.3691, 71.2613) (76.8713, 71.4272) (74.9426, 70.888) knots 0 0 0 0 1 1 1 1
  spline S260 degree 3 poles (74.9426, 70.888) (74.1338, 70.6599) (72.9102, 70.4732) (72.2466, 70.4732) knots 0 0 0 0 1 1 1 1
  spline S261 degree 3 poles (72.2466, 70.4732) (69.9239, 70.4732) (68.1196, 71.9664) (67.8085, 74.1025) knots 0 0 0 0 1 1 1 1
  spline S262 degree 3 poles (67.8085, 74.1025) (67.7256, 74.7661) (67.5182, 75.2431) (67.2486, 75.4713) knots 0 0 0 0 1 1 1 1
  spline S263 degree 3 poles (67.2486, 75.4713) (67.0205, 75.6579) (66.6887, 76.2593) (66.502, 76.8193) knots 0 0 0 0 1 1 1 1
  spline S264 degree 3 poles (66.502, 76.8193) (66.2324, 77.6073) (66.0458, 77.8355) (65.5895, 77.9599) knots 0 0 0 0 1 1 1 1
  spline S265 degree 3 poles (65.5895, 77.9599) (65.2577, 78.0636) (64.7807, 78.3125) (64.5318, 78.5613) knots 0 0 0 0 1 1 1 1
  line L20 (64.5318, 78.5613) -> (64.0756, 78.9761)
  line L21 (64.0756, 78.9761) -> (63.8475, 78.1673)
  spline S266 degree 3 poles (44.5398, 70.8673) (44.0628, 69.7681) (43.5029, 67.7565) (43.2747, 66.2011) knots 0 0 0 0 1 1 1 1
  spline S267 degree 3 poles (43.2747, 66.2011) (42.9844, 64.3553) (43.254, 62.0534) (44.0421, 59.7306) knots 0 0 0 0 1 1 1 1
  spline S268 degree 3 poles (44.0421, 59.7306) (44.7887, 57.4909) (45.5767, 56.1636) (47.0077, 54.8571) knots 0 0 0 0 1 1 1 1
  spline S269 degree 3 poles (47.0077, 54.8571) (48.1898, 53.7579) (50.8236, 52.2232) (51.0725, 52.4928) knots 0 0 0 0 1 1 1 1
  spline S270 degree 3 poles (51.0725, 52.4928) (51.1347, 52.5551) (50.948, 53.2394) (50.637, 53.986) knots 0 0 0 0 1 1 1 1
  spline S271 degree 3 poles (50.637, 53.986) (50.1185, 55.3133) (49.6, 57.4909) (49.1023, 60.5602) knots 0 0 0 0 1 1 1 1
  spline S272 degree 3 poles (49.1023, 60.5602) (48.7912, 62.4059) (47.9824, 65.1642) (47.0699, 67.5698) knots 0 0 0 0 1 1 1 1
  spline S273 degree 3 poles (47.0699, 67.5698) (46.3233, 69.4985) (45.2449, 71.5102) (44.9753, 71.5102) knots 0 0 0 0 1 1 1 1
  spline S274 degree 3 poles (44.9753, 71.5102) (44.8923, 71.5102) (44.7057, 71.2198) (44.5398, 70.8673) knots 0 0 0 0 1 1 1 1
  circle A0 centre (71.2861, 71.324) radius 43.4137
extrude "Extrude1" add sketch "Sketch1" along normal blind 25 contours A0